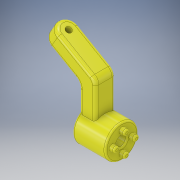
# Autodesk Inventor part: Link1
Saved by Autodesk Inventor 2019 (Build 230136000, 136)
## iProperties
Created: 2022-07-14
Part Number: Link1
Material: Generic
Document SubType Name: Modeling
Designer: zreik
Density: 1 g/cm^3
Appearance: Yellow
thickness: 10.000 mm
width: 12.000 mm
radius: 60.000 mm
Author: zreik
Autodesk Inventor part; units mm, degrees
sketch "Sketch1" plane through (0, 0, 0) normal (0, 0, 1) x (1, 0, 0)
  line L0 (46.9504, 0) -> (0, 0)
  line L1 (0, 0) -> (30, 51.9615)
  line L2 (36.9504, 0) -> (36.9504, 21.1132)
  line L3 (34.4504, 25.4434) -> (19.6299, 34)
  line L4 (46.9504, 0) -> (46.9504, 26.8868)
  line L5 (44.4504, 31.2169) -> (24.6299, 42.6603)
  arc A0 (36.9504, 21.1132) -> (34.4504, 25.4434) centre (31.9504, 21.1132) ccw
  arc A1 (46.9504, 26.8868) -> (44.4504, 31.2169) centre (41.9504, 26.8868) ccw
  line L6 (24.6299, 42.6603) -> (19.6299, 34)
  line L7 (24.6299, 42.6603) -> (44.4504, 31.2169)
  line L8 (19.6299, 34) -> (34.4504, 25.4434)
  line L9 (36.9504, 0) -> (46.9504, 0)
  line L10 (46.9504, 0) -> (46.9504, 26.8868)
  line L11 (36.9504, 0) -> (46.9504, 0)
  line L12 (46.9504, 0) -> (46.9504, 26.8868)
  line L13 (44.4504, 31.2169) -> (24.6299, 42.6603)
  line L14 (24.6299, 42.6603) -> (19.6299, 34)
  line L15 (19.6299, 34) -> (34.4504, 25.4434)
  line L16 (36.9504, 21.1132) -> (36.9504, 0)
  point P0 (25, 43.3013)
  point P1 (36.9504, 24)
  dimension "d0" = 60
  dimension "d35" = 10
  dimension "d37" = 10
  dimension "d38" = 0
  dimension "d39" = 0
  dimension "d41" = 24
  dimension "d42" = 20
  dimension "d43" = 120
  dimension "d44" = 5
  constraints: 34 end point, 9 collinear, 6 point on line, 4 point on circle, 4 tangent, 2 centre point, 2 parallel, 1 equal radius, 1 horizontal, 1 vertical
  measures "d0" angle of L1 L0
  measures "d35" distance between parallel lines of L3 L5
  measures "d37" distance between parallel lines of L4 L2
  measures "d38" distance from line of L1 L3.end
  measures "d39" distance from line of L1 L5.end
  measures "d41" distance of L2.start point (36.95, 24)
  measures "d42" distance of point (36.95, 24) L3.end
  measures "d43" angle of L2 L3
  measures "d44" radius of A0
extrude "Extrusion1" add sketch "Sketch1" along normal blind 12 contours L0 L2 A0 L3 L1 L5 A1 L4
ref_plane "Work Plane1" through (34.5402, 36.9386, 0) normal (0.5, 0.8660254, 0) x (0.8660254, -0.5, 0)
sketch "Sketch2" plane through (34.5402, 36.9386, 0) normal (0.5, 0.8660254, 0) x (0.8660254, -0.5, 0)
  circle A0 centre (-11.4434, -6) radius 6
  line L0 (-11.4434, 0) -> (-11.4434, -12) projected
  line L1 (11.4434, 0) -> (-11.4434, 0) projected
  dimension "d5" = 12
  dimension "d45" = 0
  dimension "d46" = 6
  constraints: 1 centre point
  measures "d5" diameter of A0
  measures "d45" distance from line of L0 A0.centre
  measures "d46" distance from line of L1 A0.centre
extrude "Extrusion2" add sketch "Sketch2" against normal blind 10
ref_plane "Work Plane2" through (46.9504, 0, 6) normal (1, 0, 0) x (0, 0, -1)
sketch "Sketch3" plane through (46.9504, 0, 6) normal (1, 0, 0) x (0, 0, -1)
  circle A0 centre (0, 0) radius 6
  line L0 (6, 0) -> (-6, 0) projected
  line L1 (-6, 0) -> (-6, 26.8868) projected
  point P0 (-6, 34)
  dimension "d10" = 12
  dimension "d47" = 0
  dimension "d48" = 6
  constraints: 1 centre point, 1 vertical alignment
  measures "d10" diameter of A0
  measures "d47" distance from line of L0 A0.centre
  measures "d48" distance from line of L1 A0.centre
extrude "Extrusion3" add sketch "Sketch3" against normal blind 10
sketch "Sketch4" plane through (29.5402, 28.2783, 0) normal (-0.5, -0.8660254, 0) x (-0.8660254, 0.5, 0)
  circle A0 centre (11.4434, -6) radius 1.75
  circle A1 centre (11.4434, -6) radius 6 projected
  point P0 (11.4434, 0)
  point P1 (11.4434, -12)
  dimension "d15" = 3.5
  constraints: 1 centre point, 1 concentric
  measures "d15" diameter of A0
extrude "Extrusion4" cut sketch "Sketch4" against normal blind 50 contours A0
sketch "Sketch5" plane through (36.9504, 0, 6) normal (-1, 0, 0) x (0, 1, 0)
  circle A0 centre (0, 0) radius 1.75
  arc A1 (0, 6) -> (0, -6) centre (0, 0) ccw projected
  dimension "d18" = 3.5
  constraints: 1 centre point, 1 concentric
  measures "d18" diameter of A0
extrude "Extrusion5" cut sketch "Sketch5" against normal blind 50
sketch "Sketch6" plane through (29.5402, 28.2783, 0) normal (-0.5, -0.8660254, 0) x (-0.8660254, 0.5, 0)
  circle A0 centre (11.4434, -6) radius 3.5
  circle A1 centre (11.4434, -6) radius 6 projected
  circle A2 centre (11.4434, -6) radius 1.25
  arc A3 (13.1934, -6) -> (13.1934, -6) centre (11.4434, -6) ccw projected
  point P0 (11.4434, 0)
  point P1 (11.4434, -12)
  dimension "d21" = 7
  dimension "d24" = 3
  constraints: 2 centre point, 1 coincident, 1 concentric
  measures "d21" diameter of A0
extrude "Extrusion6" add sketch "Sketch6" along normal blind 1.547 contours A0 | A3
chamfer "Chamfer1" distance 1 angle 45 1 edges at (21.8875, 30.9103, 6)
sketch "Sketch7" plane through (36.9504, 0, 6) normal (-1, 0, 0) x (0, 1, 0)
  circle A0 centre (0, 0) radius 1.5
  circle A1 centre (0, 0) radius 3.5
  arc A2 (1.75, 0) -> (1.75, 0) centre (0, 0) ccw projected
  point P0 (0, 6)
  dimension "d28" = 3
  dimension "d29" = 7
  constraints: 2 centre point, 1 coincident, 1 concentric
  measures "d28" diameter of A0
  measures "d29" diameter of A1
extrude "Extrusion7" add sketch "Sketch7" along normal blind 2.887 contours A1 | A2
chamfer "Chamfer2" distance 1 angle 45 1 edges at (34.0634, -3.5, 6)
fillet "Fillet1" radius 2 8 edges at (36.2805, 23.6132, 12) (36.9504, 10.5566, 12) (36.9504, -6, 6) (36.9504, 10.5566, 0) (36.2805, 23.6132, 0) (27.0402, 29.7217, 0) (14.4338, 37, 6) (27.0402, 29.7217, 12)
ref_plane "Work Plane3" through (0, 0, 6) normal (0, 0, 1) x (1, 0, 0)
fillet "Fillet4" radius 2 7 edges at (19.4338, 45.6603, 6) (34.5402, 36.9386, 0) (46.2805, 29.3868, 0) (46.9504, 13.4434, 0) (46.2805, 29.3868, 12) (46.9504, 13.4434, 12) (34.5402, 36.9386, 12)
sketch "Sketch10" plane through (46.9504, 0, 2) normal (1, 0, 0) x (0, 0, -1)
  circle A0 centre (-4, 0) radius 10
  circle A1 centre (-4, 0) radius 1.75 projected
  circle A2 centre (-4, 6) radius 1.75
  circle A3 centre (-10, 0) radius 1.75
  circle A4 centre (-4, -6) radius 1.75
  circle A5 centre (2, 0) radius 1.75
  point P0 (2, 0)
  dimension "d75" = 20
  dimension "d76" = 0
  dimension "d77" = 6
  dimension "d78" = 3.5
  dimension "d81" = 360
  constraints: 5 centre point, 1 concentric, 9 other
  measures "d75" diameter of A0
  measures "d76" horizontal distance of A2.centre A0.centre
  measures "d77" distance of A0.centre A2.centre
  measures "d78" diameter of A2
extrude "Extrusion9" add sketch "Sketch10" along normal mid plane 20
extrude "Extrusion10" add sketch "Sketch10" along normal blind 13 contours A2 | A3 | A4 | A5
fillet "Fillet5" [suppressed]
fillet "Fillet6" radius 1 4 edges at (59.9504, 6, 7.75) (59.9504, 0, 1.75) (59.9504, 0, 13.75) (59.9504, -6, 7.75)
fillet "Fillet7" radius 1 3 edges at (36.9504, 5.4772, -2.3666) (36.9504, -8.3666, 11.4772) (56.9504, 0, 16)
sketch "Sketch11" plane through (56.9504, 0, 6) normal (1, 0, 0) x (0, 0, -1)
  circle A0 centre (0, 0) radius 3
  circle A1 centre (0, 0) radius 1.75 projected
  point P0 (6, 0)
  dimension "d90" = 6
  constraints: 1 centre point, 1 concentric
  measures "d90" diameter of A0
extrude "Extrusion11" cut sketch "Sketch11" against normal blind 5
fillet "Fillet8" radius 1 1 edges at (56.9504, 0, 9)
equation "\"d35\" = thickness"
equation "\"d37\" = thickness"
equation "\"d3\" = width"
equation "\"d5\" = width"
equation "\"d46\" = 0.5 * width"
equation "\"d8\" = thickness"
equation "\"d10\" = width"
equation "\"d48\" = 0.5 * width"
equation "\"d13\" = thickness"
equation "\"thickness\" = 10"
equation "\"width\" = 12"
equation "\"radius\" = 60"
body "Solid1"
